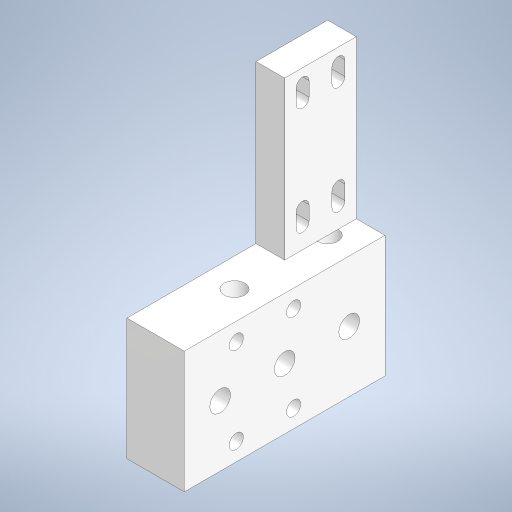
# Autodesk Inventor part: Z_probe_holder
Saved by Autodesk Inventor 2024.1 (Build 281209000, 209)
## iProperties
Created: 2023-10-06
Part Number: Z_probe_holder
Material: Generic
Document SubType Name: Modeling
Designer: l1534
Density: 1 g/cm^3
Appearance: White
Author: l1534
Autodesk Inventor part; units mm, degrees
ref_plane "YZ Plane" through (0, 0, 0) normal (1, 0, 0) x (0, 1, 0)
ref_plane "XZ Plane" through (0, 0, 0) normal (0, 1, 0) x (-1, 0, 0)
ref_plane "XY Plane" through (0, 0, 0) normal (0, 0, 1) x (1, 0, 0)
sketch "Sketch1" plane through (0, 0, 0) normal (1, 0, 0) x (0, 1, 0)
  line L0 (3.2139, -35.6679) -> (20.2139, -35.6679)
  line L1 (20.2139, -35.6679) -> (20.2139, -63.6679)
  line L2 (20.2139, -63.6679) -> (3.2139, -63.6679)
  line L3 (3.2139, -63.6679) -> (3.2139, -35.6679)
  point P0 (0, 0)
  dimension "d0" = 17
  dimension "d1" = 28
  constraints: 8 end point, 2 parallel, 1 horizontal, 1 perpendicular
  measures "d0" distance of L0.start L0.end
  measures "d1" distance of L0.end L1.end
extrude "Extrusion1" add sketch "Sketch1" along normal blind 8
sketch "Sketch2" plane through (8, 0, 0) normal (1, 0, 0) x (0, 0, -1)
  line L0 (63.6679, 3.2139) -> (63.6679, 20.2139) projected
  line L1 (63.6679, 20.2139) -> (53.6679, 20.2139)
  line L2 (53.6679, 20.2139) -> (53.6679, 42.2139)
  line L3 (53.6679, 42.2139) -> (63.6679, 42.2139)
  line L4 (63.6679, 42.2139) -> (63.6679, 20.2139)
  point P0 (0, 0)
  dimension "d4" = 10
  dimension "d5" = 22
  constraints: 8 end point, 2 parallel, 1 horizontal, 1 perpendicular
  measures "d4" distance of L2.end L3.end
  measures "d5" distance of L1.end L2.end
extrude "Extrusion2" add sketch "Sketch2" against normal up to surface (8 mm away)
sketch "Sketch3" plane through (8, 20.2139, -53.6679) normal (0, 0, 1) x (1, 0, 0)
  line L0 (-8, 0) -> (0, 0) projected
  line L1 (-8, -17) -> (-8, 22) projected
  line L2 (-4, 0) -> (-8, 0)
  line L3 (-8, 0) -> (-8, 22)
  line L4 (-8, 22) -> (-4, 22)
  line L5 (-4, 22) -> (-4, 0)
  point P0 (-8, -20.2139)
  dimension "d8" = 4
  constraints: 8 end point, 2 parallel, 1 horizontal, 1 midpoint, 1 perpendicular
  measures "d8" distance between parallel lines of L1 L5
extrude "Extrusion3" cut sketch "Sketch3" against normal through all
sketch "Sketch4" plane through (8, 0, 0) normal (1, 0, 0) x (0, 0, -1)
  circle A0 centre (42.9179, 5.7139) radius 1
  circle A1 centre (42.9179, 17.7139) radius 1
  circle A2 centre (50.9179, 5.7139) radius 1
  circle A3 centre (50.9179, 17.7139) radius 1
  line L0 (35.6679, 3.2139) -> (63.6679, 3.2139) projected
  line L1 (53.6679, 20.2139) -> (35.6679, 20.2139) projected
  line L2 (35.6679, 20.2139) -> (35.6679, 3.2139) projected
  point P0 (0, 0)
  dimension "d11" = 2
  dimension "d13" = 2
  dimension "d14" = 2
  dimension "d15" = 2
  dimension "d16" = 2.5
  dimension "d17" = 2.5
  dimension "d18" = 2.5
  dimension "d19" = 2.5
  dimension "d20" = 7.25
  dimension "d21" = 7.25
  dimension "d22" = 8
  dimension "d23" = 8
  constraints: 4 centre point
  measures "d11" diameter of A2
  measures "d13" diameter of A1
  measures "d14" diameter of A3
  measures "d15" diameter of A0
  measures "d16" distance from line of L0 A0.centre
  measures "d17" distance from line of L1 A1.centre
  measures "d18" distance from line of L1 A3.centre
  measures "d19" distance from line of L0 A2.centre
  measures "d20" distance from line of L2 A0.centre
  measures "d21" distance from line of L2 A1.centre
  measures "d22" distance of A0.centre A2.centre
  measures "d23" distance of A1.centre A3.centre
extrude "Extrusion4" cut sketch "Sketch4" against normal through all
sketch "Sketch5" plane through (0, 3.2139, -63.6679) normal (0, -1, 0) x (1, 0, 0)
  line L0 (4, 10) -> (4, 0) projected
  circle A0 centre (4, 4) radius 1.45
  circle A1 centre (4, 17) radius 1.45
  line L1 (8, 28) -> (8, 0) projected
  line L2 (0, 0) -> (8, 0) projected
  point P0 (0, 63.6679)
  dimension "d26" = 2.9
  dimension "d27" = 2.9
  dimension "d28" = 4
  dimension "d29" = 4
  dimension "d30" = 17
  constraints: 2 centre point, 1 point on line
  measures "d26" diameter of A1
  measures "d27" diameter of A0
  measures "d28" distance from line of L1 A1.centre
  measures "d29" distance from line of L2 A0.centre
  measures "d30" distance from line of L2 A1.centre
extrude "Extrusion5" cut sketch "Sketch5" against normal up to surface (17 mm away)
chamfer "Chamfer1" distance 0.2 angle 45 2 edges at (2.55, 3.2139, -46.6679) (2.55, 3.2139, -59.6679)
sketch "Sketch8" plane through (8, 0, 0) normal (1, 0, 0) x (0, 0, -1)
  circle A0 centre (40.6679, 11.7139) radius 1.45
  circle A1 centre (58.6679, 11.7139) radius 1.45
  circle A2 centre (49.6679, 11.7139) radius 1.45
  line L0 (53.6679, 20.2139) -> (35.6679, 20.2139) projected
  line L1 (35.6679, 3.2139) -> (63.6679, 3.2139) projected
  line L2 (63.6679, 3.2139) -> (63.6679, 42.2139) projected
  line L3 (35.6679, 20.2139) -> (35.6679, 3.2139) projected
  point P0 (0, 0)
  dimension "d53" = 8.5
  dimension "d54" = 8.5
  dimension "d55" = 8.5
  dimension "d56" = 2.9
  dimension "d57" = 2.9
  dimension "d58" = 2.9
  dimension "d59" = 5
  dimension "d60" = 14
  dimension "d61" = 5
  constraints: 3 centre point
  measures "d53" distance from line of L0 A0.centre
  measures "d54" distance from line of L0 A2.centre
  measures "d55" distance from line of L1 A1.centre
  measures "d56" diameter of A0
  measures "d57" diameter of A2
  measures "d58" diameter of A1
  measures "d59" distance from line of L2 A1.centre
  measures "d60" distance from line of L2 A2.centre
  measures "d61" distance from line of L3 A0.centre
extrude "Extrusion7" cut sketch "Sketch8" against normal through all
chamfer "Chamfer3" distance 1.4 angle 45 4 edges at (8, 5.7139, -41.9179) (8, 17.7139, -41.9179) (8, 17.7139, -49.9179) (8, 5.7139, -49.9179)
sketch "Sketch9" plane through (8, 0, 0) normal (1, 0, 0) x (0, 0, -1)
  circle A0 centre (56.1679, 25.2139) radius 0.9
  circle A1 centre (61.1679, 25.2139) radius 0.9
  circle A2 centre (61.1679, 40.2139) radius 0.9
  circle A3 centre (56.1679, 40.2139) radius 0.9
  line L0 (53.6679, 42.2139) -> (53.6679, 20.2139) projected
  line L1 (63.6679, 42.2139) -> (53.6679, 42.2139) projected
  line L2 (63.6679, 3.2139) -> (63.6679, 42.2139) projected
  line L3 (55.2679, 25.2139) -> (57.0679, 25.2139)
  line L4 (57.0679, 25.2139) -> (57.0679, 23.2139)
  line L5 (57.0679, 23.2139) -> (55.2679, 23.2139)
  line L6 (55.2679, 23.2139) -> (55.2679, 25.2139)
  line L7 (60.2679, 25.2139) -> (62.0679, 25.2139)
  line L8 (62.0679, 25.2139) -> (62.0679, 23.2139)
  line L9 (62.0679, 23.2139) -> (60.2679, 23.2139)
  line L10 (60.2679, 23.2139) -> (60.2679, 25.2139)
  line L11 (57.0679, 40.2139) -> (55.2679, 40.2139)
  line L12 (55.2679, 40.2139) -> (55.2679, 38.2139)
  line L13 (55.2679, 38.2139) -> (57.0679, 38.2139)
  line L14 (57.0679, 38.2139) -> (57.0679, 40.2139)
  line L15 (62.0679, 40.2139) -> (60.2679, 40.2139)
  line L16 (60.2679, 40.2139) -> (60.2679, 38.2139)
  line L17 (60.2679, 38.2139) -> (62.0679, 38.2139)
  line L18 (62.0679, 38.2139) -> (62.0679, 40.2139)
  arc A4 (55.2679, 23.2139) -> (57.0679, 23.2139) centre (56.1679, 23.2139) ccw
  arc A5 (60.2679, 23.2139) -> (62.0679, 23.2139) centre (61.1679, 23.1946) ccw
  arc A6 (60.2679, 38.2139) -> (62.0679, 38.2139) centre (61.1679, 38.2139) ccw
  arc A7 (55.2679, 38.2139) -> (57.0679, 38.2139) centre (56.1679, 38.2139) ccw
  point P0 (0, 0)
  dimension "d70" = 1.8
  dimension "d71" = 1.8
  dimension "d72" = 1.8
  dimension "d73" = 1.8
  dimension "d74" = 2.5
  dimension "d75" = 2
  dimension "d76" = 2
  dimension "d77" = 2.5
  dimension "d78" = 2.5
  dimension "d79" = 2.5
  dimension "d80" = 15
  dimension "d81" = 15
  dimension "d82" = 1.8
  dimension "d83" = 1.8
  dimension "d84" = 1.8
  dimension "d85" = 2
  dimension "d86" = 2
  dimension "d87" = 2
  dimension "d88" = 0.9
  dimension "d89" = 0.9
  constraints: 32 end point, 8 parallel, 8 point on circle, 4 centre point, 4 horizontal, 4 perpendicular, 4 point on line, 2 tangent, 12 other
  measures "d74" distance from line of L0 point (56.168, 40.214)
  measures "d75" distance from line of L1 point (56.168, 40.214)
  measures "d76" distance from line of L1 point (61.168, 40.214)
  measures "d77" distance from line of L2 point (61.168, 40.214)
  measures "d78" distance from line of L0 point (56.168, 25.214)
  measures "d79" distance from line of L2 point (61.168, 25.214)
  measures "d80" distance of point (61.168, 40.214) point (61.168, 25.214)
  measures "d81" distance of point (56.168, 40.214) point (56.168, 25.214)
  measures "d82" distance of L16.end L17.end
  measures "d83" distance of L12.end L13.end
  measures "d84" distance of L8.end L9.end
  measures "d85" distance of L9.end L7.start
  measures "d86" distance of L11.end L12.end
  measures "d87" distance of L15.end L16.end
  measures "d88" radius of A6
  measures "d89" radius of A7
extrude "Extrusion8" cut sketch "Sketch9" against normal through all
mirror "Mirror1" about plane through (8, 11.7139, -49.6679) normal (1, 0, 0) remove original yes
body "Solid1"
